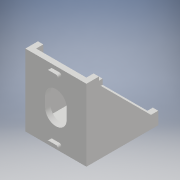
# Autodesk Inventor part: 90 angle
Saved by Autodesk Inventor 2018 (Build 220112000, 112)
## iProperties
Created: 2018-05-23
Part Number: 90 angle
Material: Generic
Document SubType Name: Modeling
Designer: Z. Deniz
Density: 1 g/cm^3
Appearance: Default
Author: Z. Deniz
Autodesk Inventor part; units mm, degrees
ref_plane "YZ Plane" through (0, 0, 0) normal (1, 0, 0) x (0, 1, 0)
ref_plane "XZ Plane" through (0, 0, 0) normal (0, 1, 0) x (-1, 0, 0)
ref_plane "XY Plane" through (0, 0, 0) normal (0, 0, 1) x (1, 0, 0)
sketch "Sketch1" plane through (0, 0, 0) normal (0, 0, 1) x (1, 0, 0)
  line L0 (-8.5, 10) -> (8.5, 10)
  line L1 (8.5, 10) -> (8.5, -10)
  line L2 (8.5, -10) -> (-8.5, -10)
  line L3 (-8.5, -10) -> (-8.5, 10)
  line L4 (-8.5, 10) -> (8.5, -10) construction
  line L5 (8.5, 10) -> (-8.5, -10) construction
  line L6 (0, 1.5) -> (0, -1.5) construction
  line L7 (-3, 1.5) -> (-3, -1.5)
  line L8 (3, -1.5) -> (3, 1.5)
  arc A0 (3, 1.5) -> (-3, 1.5) centre (0, 1.5) ccw
  arc A1 (-3, -1.5) -> (3, -1.5) centre (0, -1.5) ccw
  line L9 (-1, -8.5) -> (1, -8.5) construction
  line L10 (-1, -9) -> (1, -9)
  line L11 (1, -8) -> (-1, -8)
  arc A2 (-1, -8) -> (-1, -9) centre (-1, -8.5) ccw
  arc A3 (1, -9) -> (1, -8) centre (1, -8.5) ccw
  line L12 (-8.5, 0) -> (8.5, 0) construction
  line L13 (-1, 8.5) -> (1, 8.5) construction
  line L14 (-1, 9) -> (1, 9)
  line L15 (1, 8) -> (-1, 8)
  arc A4 (-1, 9) -> (-1, 8) centre (-1, 8.5) ccw
  arc A5 (1, 8) -> (1, 9) centre (1, 8.5) ccw
  line L16 (7, -10) -> (7, 10)
  line L17 (-7, -10) -> (-7, 10)
  line L18 (-8.5, -8.5) -> (-7, -8.5)
  line L19 (7, -8.5) -> (8.5, -8.5)
  line L20 (-7, -8.5) -> (7, -8.5)
  point P0 (0, 0)
  point P1 (0, -8.5)
  point P2 (0, 8.5)
  dimension "d0" = 17
  dimension "d1" = 20
  dimension "d2" = 1.5
  dimension "d3" = 6
  dimension "d4" = 1
  dimension "d5" = 1
  dimension "d6" = 1.5
  dimension "d7" = 8.5
  dimension "d37" = 1.5
  dimension "d38" = 1.5
  dimension "d41" = 1.5
  constraints: 48 end point, 12 point on circle, 8 point on line, 8 tangent, 7 symmetric about line, 6 centre point, 6 midpoint, 6 perpendicular, 4 parallel, 2 horizontal, 1 vertical, 2 other
  measures "d0" distance of L1.end L2.end
  measures "d1" distance of L0.end L1.end
  measures "d2" distance of point (0, 0) L6.end
  measures "d3" diameter of A1
  measures "d4" distance of point (0, -8.5) L9.end
  measures "d5" diameter of A3
  measures "d6" distance from line of L2 point (0, -8.5)
  measures "d7" distance from line of L1 point (0, -8.5)
  measures "d37" distance between parallel lines of L1 L16
  measures "d38" distance between parallel lines of L17 L3
  measures "d41" distance between parallel lines of L2 L18
extrude "Extrusion5" add sketch "Sketch1" along normal blind 20 contours L0 L17 L18 L3 | L18 L17 L2 L3 | L0 L1 L19 L16 | L20 A2 L10 A3 L16 L2 L17 | L19 L1 L2 L16 | L20 A3 L10 A2
extrude "Extrusion6" add sketch "Sketch1" along normal blind 2 contours L0 L16 L20 A3 L11 A2 L17 | A2 L11 A3 L20
extrude "Extrusion7" add sketch "Sketch1" along normal blind 2 and the other way blind 1 contours L20 A3 L10 A2 | A2 L11 A3 L20 | L14 A5 L15 A4
sketch "Sketch8" plane through (-8.5, -10, 0) normal (0, -1, 0) x (1, 0, 0)
  line L0 (0, 20) -> (17, 20)
  line L1 (17, 20) -> (17, 0)
  line L2 (17, 0) -> (0, 0)
  line L3 (0, 0) -> (0, 20)
  line L4 (0, 20) -> (17, 0) construction
  line L5 (17, 20) -> (0, 0) construction
  line L6 (8.5, 11.5) -> (8.5, 8.5) construction
  line L7 (5.5, 11.5) -> (5.5, 8.5)
  line L8 (11.5, 8.5) -> (11.5, 11.5)
  arc A0 (11.5, 11.5) -> (5.5, 11.5) centre (8.5, 11.5) ccw
  arc A1 (5.5, 8.5) -> (11.5, 8.5) centre (8.5, 8.5) ccw
  line L9 (7.5, 1.5) -> (9.5, 1.5) construction
  line L10 (7.5, 1) -> (9.5, 1)
  line L11 (9.5, 2) -> (7.5, 2)
  arc A2 (7.5, 2) -> (7.5, 1) centre (7.5, 1.5) ccw
  arc A3 (9.5, 1) -> (9.5, 2) centre (9.5, 1.5) ccw
  line L12 (0, 10) -> (17, 10) construction
  arc A4 (7.5, 19) -> (7.5, 18) centre (7.5, 18.5) ccw
  line L13 (7.5, 18.5) -> (9.5, 18.5) construction
  line L14 (7.5, 19) -> (9.5, 19)
  line L15 (9.5, 18) -> (7.5, 18)
  arc A5 (9.5, 18) -> (9.5, 19) centre (9.5, 18.5) ccw
  line L16 (15.5, 0) -> (15.5, 20)
  line L17 (1.5, 0) -> (1.5, 20)
  line L18 (0, 1.5) -> (1.5, 1.5)
  line L19 (15.5, 1.5) -> (17, 1.5)
  line L20 (1.5, 1.5) -> (15.5, 1.5)
  line L21 (17, 0) -> (17, 20) projected
  line L22 (0, 20) -> (17, 20) projected
  point P0 (8.5, 0)
  point P1 (8.5, 10)
  point P2 (8.5, 1.5)
  point P3 (8.5, 18.5)
  dimension "d66" = 17
  dimension "d67" = 20
  dimension "d68" = 1.5
  dimension "d69" = 6
  dimension "d70" = 1
  dimension "d71" = 1
  dimension "d72" = 1.5
  dimension "d73" = 8.5
  dimension "d74" = 1.5
  dimension "d75" = 1.5
  dimension "d76" = 1.5
  constraints: 48 end point, 12 point on circle, 8 point on line, 8 tangent, 7 symmetric about line, 6 centre point, 6 midpoint, 6 perpendicular, 4 parallel, 2 collinear, 2 horizontal, 1 vertical, 2 other
  measures "d66" distance of L1.end L2.end
  measures "d67" distance of L0.end L1.end
  measures "d68" distance of point (8.5, 10) L6.end
  measures "d69" diameter of A1
  measures "d70" distance of point (8.5, 1.5) L9.end
  measures "d71" diameter of A3
  measures "d72" distance from line of L2 point (8.5, 1.5)
  measures "d73" distance from line of L1 point (8.5, 1.5)
  measures "d74" distance between parallel lines of L1 L16
  measures "d75" distance between parallel lines of L17 L3
  measures "d76" distance between parallel lines of L2 L18
extrude "Extrusion9" cut sketch "Sketch8" against normal blind 2 contours A0 L8 A1 L7
extrude "Extrusion10" add sketch "Sketch8" along normal blind 1 and the other way blind 2 contours L20 A3 L10 A2 | A2 L11 A3 L20 | L14 A5 L15 A4
sketch "Sketch9" plane through (-8.5, 10, 0) normal (0, 1, 0) x (1, 0, 0)
  line L0 (1.5, -2) -> (1.5, -20) projected
  line L1 (1.5, -20) -> (0, -20)
  line L2 (0, -20) -> (0, -3.5)
  line L3 (0, -3.5) -> (1.5, -3.5)
  line L4 (1.5, -3.5) -> (1.5, -20)
  line L5 (17, -20) -> (15.5, -20) projected
  line L6 (17, -20) -> (15.5, -20)
  line L7 (15.5, -20) -> (15.5, -3.5)
  line L8 (15.5, -3.5) -> (17, -3.5)
  line L9 (17, -3.5) -> (17, -20)
  point P0 (8.5, 0)
  dimension "d83" = 1.5
  dimension "d84" = 16.5
  dimension "d85" = 1.5
  dimension "d86" = 16.5
  constraints: 16 end point, 4 parallel, 2 horizontal, 2 perpendicular
  measures "d83" distance of L2.end L3.end
  measures "d84" distance of L1.end L2.end
  measures "d85" distance of L7.end L8.end
  measures "d86" distance of L6.end L7.end
sketch "Sketch10" plane through (0, 0, 20) normal (0, 0, 1) x (1, 0, 0)
  line L0 (8.5, -10) -> (8.5, 10) projected
  line L1 (8.5, 10) -> (7, 10)
  line L2 (7, 10) -> (7, -6.5)
  line L3 (7, -6.5) -> (8.5, -6.5)
  line L4 (8.5, -6.5) -> (8.5, 10)
  line L5 (-7, 10) -> (-8.5, 10) projected
  line L6 (-7, -8.5) -> (-7, 10) projected
  line L7 (-8.5, 10) -> (-7, 10)
  line L8 (-7, 10) -> (-7, -6.5)
  line L9 (-7, -6.5) -> (-8.5, -6.5)
  line L10 (-8.5, -6.5) -> (-8.5, 10)
  point P0 (0, 0)
  dimension "d87" = 1.5
  dimension "d88" = 16.5
  dimension "d89" = 16.5
  constraints: 16 end point, 4 parallel, 2 horizontal, 2 perpendicular, 1 point on line
  measures "d87" distance of L3.end L2.end
  measures "d88" distance of L2.end L1.end
  measures "d89" distance of L7.end L8.end
extrude "Extrusion11" cut sketch "Sketch9" against normal blind 2
extrude "Extrusion12" cut sketch "Sketch10" against normal blind 2
chamfer "Chamfer3" distance 14.5 angle 45 1 edges at (-7.75, 8, 18)
chamfer "Chamfer4" distance 14.5 angle 45 1 edges at (7.75, 8, 18)
body "Solid2"
